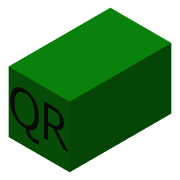
# Autodesk Inventor part: Container 2 2 2 and half color 2
Saved by Autodesk Inventor 2015 (Build 190159000, 159)
## iProperties
Created: 2015-03-07
Part Number: Container 2 2 2 and half color 2
Material: Generic
Document SubType Name: Modeling
Designer: Vukica
Density: 1 g/cm^3
Appearance: Dark Green
Author: Vukica
Autodesk Inventor part; units mm, degrees
ref_plane "YZ Plane" through (0, 0, 0) normal (1, 0, 0) x (0, 1, 0)
ref_plane "XZ Plane" through (0, 0, 0) normal (0, 1, 0) x (-1, 0, 0)
ref_plane "XY Plane" through (0, 0, 0) normal (0, 0, 1) x (1, 0, 0)
sketch "Sketch1" plane through (0, 0, 0) normal (0, 0, 1) x (1, 0, 0)
  line L0 (0, 0) -> (38.1, 0)
  line L1 (38.1, 0) -> (38.1, 38.1)
  line L2 (38.1, 38.1) -> (0, 38.1)
  line L3 (0, 38.1) -> (0, 0)
  dimension "d0" = 38.1
  dimension "d1" = 38.1
  constraints: 8 end point, 2 parallel, 1 horizontal, 1 perpendicular
  measures "d0" distance of L1.end L2.end
  measures "d1" distance of L2.end L0.start
extrude "Extrusion1" add sketch "Sketch1" along normal blind 63.5
sketch "Sketch2" plane through (0, 0, 63.5) normal (0, 0, 1) x (1, 0, 0)
  line L0 (-0.0196, 30.7582) -> (23.178, 30.7582) construction
  line L1 (23.178, 30.7582) -> (23.178, 14.4458) construction
  line L2 (23.178, 14.4458) -> (-0.0196, 14.4458) construction
  line L3 (-0.0196, 14.4458) -> (-0.0196, 30.7582) construction
  spline S0 degree 2 poles (18.9172, 5.0371) (18.1762, 4.856) (16.5625, 4.6584) (15.7556, 4.6584) knots 0 0 0 1 2 2 2
  spline S1 degree 2 poles (15.7556, 4.6584) (13.4667, 4.6584) (10.618, 7.2107) (10.4862, 9.5819) knots 0 0 0 1 2 2 2
  spline S2 degree 2 poles (10.4862, 9.5819) (10.3051, 9.5819) (9.9922, 9.5819) (9.8605, 9.5819) knots 0 0 0 1 2 2 2
  spline S3 degree 2 poles (9.8605, 9.5819) (7.8021, 9.5819) (4.4923, 10.9816) (3.3067, 12.3484) knots 0 0 0 1 2 2 2
  spline S4 degree 2 poles (3.3067, 12.3484) (2.1376, 13.6986) (0.8861, 17.6507) (0.8861, 20.1536) knots 0 0 0 1 2 2 2
  spline S5 degree 2 poles (0.8861, 20.1536) (0.8861, 22.7224) (2.154, 26.6086) (3.3232, 27.9918) knots 0 0 0 1 2 2 2
  spline S6 degree 2 poles (3.3232, 27.9918) (4.5088, 29.3585) (7.8186, 30.7582) (9.8605, 30.7582) knots 0 0 0 1 2 2 2
  spline S7 degree 2 poles (9.8605, 30.7582) (11.9353, 30.7582) (15.2616, 29.3091) (16.4143, 27.9918) knots 0 0 0 1 2 2 2
  spline S8 degree 2 poles (16.4143, 27.9918) (17.5669, 26.658) (18.8514, 22.6895) (18.8514, 20.1536) knots 0 0 0 1 2 2 2
  spline S9 degree 2 poles (18.8514, 20.1536) (18.8514, 16.2016) (15.7721, 11.0639) (13.088, 10.1583) knots 0 0 0 1 2 2 2
  spline S10 degree 2 poles (13.088, 10.1583) (13.1538, 9.4008) (13.5491, 8.1823) (13.8619, 7.8365) knots 0 0 0 1 2 2 2
  spline S11 degree 2 poles (13.8619, 7.8365) (14.2407, 7.4083) (15.2781, 7.0131) (16.2002, 7.0131) knots 0 0 0 1 2 2 2
  spline S12 degree 2 poles (16.2002, 7.0131) (16.7436, 7.0131) (18.2256, 7.3589) (18.555, 7.4907) knots 0 0 0 1 2 2 2
  line L4 (18.555, 7.4907) -> (18.9172, 7.4907)
  line L5 (18.9172, 7.4907) -> (18.9172, 5.0371)
  spline S13 degree 2 poles (16.0355, 20.1536) (16.0355, 22.179) (15.1628, 25.2912) (14.3724, 26.3122) knots 0 0 0 1 2 2 2
  spline S14 degree 2 poles (14.3724, 26.3122) (13.5655, 27.366) (11.2931, 28.4199) (9.877, 28.4199) knots 0 0 0 1 2 2 2
  spline S15 degree 2 poles (9.877, 28.4199) (8.4114, 28.4199) (6.2049, 27.399) (5.3651, 26.3122) knots 0 0 0 1 2 2 2
  spline S16 degree 2 poles (5.3651, 26.3122) (4.5582, 25.2748) (3.7019, 22.1296) (3.7019, 20.1536) knots 0 0 0 1 2 2 2
  spline S17 degree 2 poles (3.7019, 20.1536) (3.7019, 16.1522) (7.0611, 11.8873) (9.877, 11.8873) knots 0 0 0 1 2 2 2
  spline S18 degree 2 poles (9.877, 11.8873) (12.6928, 11.8873) (16.0355, 16.1522) (16.0355, 20.1536) knots 0 0 0 1 2 2 2
  line L6 (37.5411, 10.0101) -> (34.0337, 10.0101)
  line L7 (34.0337, 10.0101) -> (27.6117, 18.0953)
  line L8 (27.6117, 18.0953) -> (24.5159, 18.0953)
  line L9 (24.5159, 18.0953) -> (24.5159, 10.0101)
  line L10 (24.5159, 10.0101) -> (21.8154, 10.0101)
  line L11 (21.8154, 10.0101) -> (21.8154, 30.3301)
  line L12 (21.8154, 30.3301) -> (27.0518, 30.3301)
  spline S19 degree 2 poles (27.0518, 30.3301) (28.7973, 30.3301) (31.152, 29.9513) (32.2224, 29.2597) knots 0 0 0 1 2 2 2
  spline S20 degree 2 poles (32.2224, 29.2597) (33.2927, 28.5681) (34.5277, 26.411) (34.5277, 24.8137) knots 0 0 0 1 2 2 2
  spline S21 degree 2 poles (34.5277, 24.8137) (34.5277, 22.5907) (32.2553, 19.5773) (30.3122, 18.8527) knots 0 0 0 1 2 2 2
  line L13 (30.3122, 18.8527) -> (37.5411, 10.0101)
  spline S22 degree 2 poles (31.7119, 24.5996) (31.7119, 25.4888) (31.0862, 26.8556) (30.4275, 27.3002) knots 0 0 0 1 2 2 2
  spline S23 degree 2 poles (30.4275, 27.3002) (29.8512, 27.6789) (28.3197, 27.9918) (27.2, 27.9918) knots 0 0 0 1 2 2 2
  line L14 (27.2, 27.9918) -> (24.5159, 27.9918)
  line L15 (24.5159, 27.9918) -> (24.5159, 20.3512)
  line L16 (24.5159, 20.3512) -> (26.8871, 20.3512)
  spline S24 degree 2 poles (26.8871, 20.3512) (28.0563, 20.3512) (29.917, 20.7629) (30.5592, 21.4051) knots 0 0 0 1 2 2 2
  spline S25 degree 2 poles (30.5592, 21.4051) (31.152, 21.9649) (31.7119, 23.5458) (31.7119, 24.5996) knots 0 0 0 1 2 2 2
  point P0 (0, 0)
  constraints: 2 other
extrude "Extrusion2" cut sketch "Sketch2" against normal blind 0.254
equation "\"d1\" = d0"
body "Solid1"
